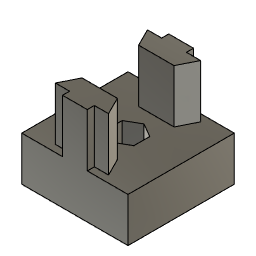
X#1slot_ext_connector (Autodesk Fusion 360 design; units mm, degrees)
Autodesk Fusion 360 part; units mm, degrees
sketch "Sketch1" plane through (0, 0, 0) normal (0, 0, 1) x (1, 0, 0)
  line L0 (0, 0) -> (30, 0)
  line L1 (30, 0) -> (30, 30)
  line L2 (30, 30) -> (0, 30)
  line L3 (0, 30) -> (0, 0)
  dimension "d1" = 30
  dimension "d2" = 30
  constraint horizontal L0
  constraint vertical L1
  constraint horizontal L2
  constraint vertical L3
  constraint coincident L0.start L3.end
  measures "d1" distance of L0.start L0.end
  measures "d2" distance of L0.start L2.end
extrude "Extrude1" add sketch "Sketch1" along normal blind 12.5
sketch "Sketch2" plane through (0, 0, 12.5) normal (0, 0, 1) x (-1, 0, 0)
  line L0 (0, -30) -> (0, 0)
  line L1 (0, 0) -> (-30, 0)
  line L2 (-30, 0) -> (-30, -30)
  line L3 (-30, -30) -> (0, -30)
  line L4 (-15, -30) -> (-11.5, -30)
  line L5 (-15, -30) -> (-18.5, -30)
  line L6 (-18.5, -30) -> (-18.5, -28)
  line L7 (-11.5, -30) -> (-11.5, -28)
  line L8 (-15, -28) -> (-22.5, -28)
  line L9 (-15, -28) -> (-7.5, -28)
  line L10 (-15, -30) -> (-15, -23)
  line L11 (-15, -23) -> (-10, -23)
  line L12 (-15, -23) -> (-20, -23)
  line L13 (-10, -23) -> (-7.5, -28)
  line L14 (-20, -23) -> (-22.5, -28)
  dimension "d5" = 3.5
  dimension "d6" = 3.5
  dimension "d7" = 7.5
  dimension "d8" = 7.5
  dimension "d9" = 7
  dimension "d10" = 5
  dimension "d11" = 5
  constraint midpoint L3 L4.start
  constraint parallel L3 L4
  constraint parallel L3 L5
  constraint perpendicular L5 L6
  constraint perpendicular L4 L7
  constraint perpendicular L6 L8
  constraint parallel L8 L9
  constraint perpendicular L9 L10
  constraint perpendicular L10 L11
  constraint perpendicular L10 L12
  measures "d5" distance of L4.start L4.end
  measures "d6" distance of L4.start L5.end
  measures "d7" distance of L8.start L8.end
  measures "d8" distance of L8.start L9.end
  measures "d9" distance of L4.start L10.end
  measures "d10" distance of L10.end L11.end
  measures "d11" distance of L10.end L12.end
extrude "Extrude2" add sketch "Sketch2" along normal blind 15 contours L3 L4 L7 L9 L10 | L3 L5 L6 L8 L10 | L9 L10 L11 L13 | L8 L10 L12 L14
sketch "Sketch3" plane through (0, 0, 12.5) normal (0, 0, 1) x (-1, 0, 0)
  line L0 (-18.5, -30) -> (-18.5, -28)
  line L1 (-18.5, -28) -> (-22.5, -28)
  line L2 (-22.5, -28) -> (-20, -23)
  line L3 (-20, -23) -> (-10, -23)
  line L4 (-10, -23) -> (-7.5, -28)
  line L5 (-7.5, -28) -> (-11.5, -28)
  line L6 (-11.5, -28) -> (-11.5, -30)
  line L7 (-11.5, -30) -> (0, -30)
  line L8 (0, -30) -> (0, 0)
  line L9 (0, 0) -> (-30, 0)
  line L10 (-30, 0) -> (-30, -30)
  line L11 (-30, -30) -> (-18.5, -30)
  line L12 (-11.5, 0) -> (-11.5, -2)
  line L13 (-18.5, 0) -> (-18.5, -2)
  line L14 (-11.5, -2) -> (-7.5, -2)
  line L15 (-18.5, -2) -> (-22.5, -2)
  line L16 (-15, 0) -> (-15, -7)
  line L17 (-15, -7) -> (-20, -7)
  line L18 (-20, -7) -> (-22.5, -2)
  line L19 (-15, -7) -> (-10, -7)
  line L20 (-7.5, -2) -> (-10, -7)
  dimension "d15" = 4
  dimension "d16" = 4
  dimension "d17" = 7
  dimension "d18" = 5
  constraint coincident L9 L12.start
  constraint perpendicular L9 L12
  constraint coincident L9 L13.start
  constraint perpendicular L12 L14
  constraint perpendicular L13 L15
  constraint midpoint L9 L16.start
  constraint perpendicular L9 L16
  constraint perpendicular L16 L17
  constraint perpendicular L16 L19
  measures "d15" distance of L12.end L14.end
  measures "d16" distance of L13.end L15.end
  measures "d17" distance of L16.start L16.end
  measures "d18" distance of L16.end L17.end
extrude "Extrude3" add sketch "Sketch3" along normal blind 15 contours L9 L13 L15 L16 L17 L18 | L9 L12 L14 L16 L19 L20
sketch "Sketch4" plane through (0, 0, 12.5) normal (0, 0, 1) x (-1, 0, 0)
  line L0 (-18.5, -2) -> (-18.5, 0)
  line L1 (-18.5, 0) -> (-30, 0)
  line L2 (-30, 0) -> (-30, -30)
  line L3 (-30, -30) -> (-18.5, -30)
  line L4 (-18.5, -30) -> (-18.5, -28)
  line L5 (-18.5, -28) -> (-22.5, -28)
  line L6 (-22.5, -28) -> (-20, -23)
  line L7 (-20, -23) -> (-10, -23)
  line L8 (-10, -23) -> (-7.5, -28)
  line L9 (-7.5, -28) -> (-11.5, -28)
  line L10 (-11.5, -28) -> (-11.5, -30)
  line L11 (-11.5, -30) -> (0, -30)
  line L12 (0, -30) -> (0, 0)
  line L13 (0, 0) -> (-11.5, 0)
  line L14 (-11.5, 0) -> (-11.5, -2)
  line L15 (-11.5, -2) -> (-7.5, -2)
  line L16 (-7.5, -2) -> (-10, -7)
  line L17 (-10, -7) -> (-20, -7)
  line L18 (-20, -7) -> (-22.5, -2)
  line L19 (-22.5, -2) -> (-18.5, -2)
  line L20 (-15, -10.5) -> (-18.8971, -12.75)
  line L21 (-18.8971, -12.75) -> (-18.8971, -17.25)
  line L22 (-18.8971, -17.25) -> (-15, -19.5)
  line L23 (-15, -19.5) -> (-11.1029, -17.25)
  line L24 (-11.1029, -17.25) -> (-11.1029, -12.75)
  line L25 (-11.1029, -12.75) -> (-15, -10.5)
  point P0 (-15, -15)
  dimension "d21" = 4.5
  measures "d21" distance of L20.start P0
extrude "Extrude4" cut sketch "Sketch4" against normal blind 6 contours L20 L21 L22 L23 L24 L25
sketch "Sketch5" plane through (0, 0, 6.5) normal (0, 0, 1) x (-1, 0, 0)
  line L0 (-11.1029, -12.75) -> (-15, -10.5)
  line L1 (-15, -10.5) -> (-18.8971, -12.75)
  line L2 (-18.8971, -12.75) -> (-18.8971, -17.25)
  line L3 (-18.8971, -17.25) -> (-15, -19.5)
  line L4 (-15, -19.5) -> (-11.1029, -17.25)
  line L5 (-11.1029, -17.25) -> (-11.1029, -12.75)
  circle A0 centre (-15, -15) radius 2.55
  dimension "d24" = 5.1
  measures "d24" diameter of A0
extrude "Extrude5" cut sketch "Sketch5" against normal blind 50 contours A0
equation "d7 = ( 15 / 2 ) * 1 mm"
equation "d21 = ( 9 / 2 ) * 1 mm"
